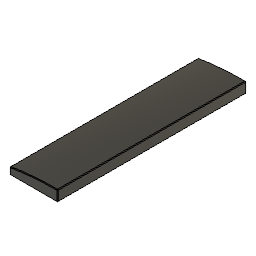
wrist_rest (Autodesk Fusion 360 design; units mm, degrees)
part number: 2026-06-30-23-31-08-090
Autodesk Fusion 360 part; units mm, degrees
sketch "Sketch1" plane through (0, 0, 0) normal (0, 0, 1) x (1, 0, 0)
  line L0 (0, 0) -> (78.5, 0)
  line L1 (0, 0) -> (0, 18)
  line L2 (78.5, 0) -> (78.5, 11.8)
  arc A0 (78.5, 11.8) -> (0, 18) centre (2.1231, -455.1742) ccw
  dimension "d3" = 78.5
  dimension "d4" = 18
  dimension "d5" = 11.8
  constraint coincident L0.start L1.start
  constraint horizontal L0
  constraint perpendicular L0 L1
  constraint perpendicular L0 L2
  measures "d3" distance of L0.start L0.end
  measures "d4" distance of L0.start L1.end
  measures "d5" distance of L0.end L2.end
extrude "Extrude1" add sketch "Sketch1" along normal blind 310
move_body "Move1" bodies 1 to x (1, 0, 0) y (0, 0, -1) z (0, 1, 0) at (0, 0, 0)
move_body "Move2" bodies 1 to x (-1, 0, 0) y (0, 1, 0) z (0, 0, -1) at (0, 0, 0)
sketch "Sketch3" plane through (0, 0, 0) normal (0, 0, -1) x (1, 0, 0)
  line L0 (0, 0) -> (-78.5, 0)
  line L1 (-78.5, 0) -> (-78.5, -310)
  line L2 (-78.5, -310) -> (0, -310)
  line L3 (0, -310) -> (0, 0)
  line L4 (-4, -306) -> (-4, -4)
  line L5 (-4, -4) -> (-74.5, -4)
  line L6 (-74.5, -4) -> (-74.5, -306)
  line L7 (-74.5, -306) -> (-4, -306)
  line L8 (-23.4372, -294.0415) -> (-16.4372, -298.0829)
  line L9 (-16.4372, -298.0829) -> (-9.4372, -294.0415)
  line L10 (-9.4372, -294.0415) -> (-9.4372, -285.9585)
  line L11 (-9.4372, -285.9585) -> (-16.4372, -281.9171)
  line L12 (-16.4372, -281.9171) -> (-23.4372, -285.9585)
  line L13 (-23.4372, -285.9585) -> (-23.4372, -294.0415)
  line L14 (-32.4372, -294.0415) -> (-32.4372, -285.9585)
  line L15 (-46.4372, -294.0415) -> (-39.4372, -298.0829)
  line L16 (-39.4372, -298.0829) -> (-32.4372, -294.0415)
  line L17 (-46.4372, -285.9585) -> (-46.4372, -294.0415)
  line L18 (-32.4372, -285.9585) -> (-39.4372, -281.9171)
  line L19 (-39.4372, -281.9171) -> (-46.4372, -285.9585)
  line L20 (-55.4372, -294.0415) -> (-55.4372, -285.9585)
  line L21 (-69.4372, -294.0415) -> (-62.4372, -298.0829)
  line L22 (-62.4372, -298.0829) -> (-55.4372, -294.0415)
  line L23 (-69.4372, -285.9585) -> (-69.4372, -294.0415)
  line L24 (-55.4372, -285.9585) -> (-62.4372, -281.9171)
  line L25 (-62.4372, -281.9171) -> (-69.4372, -285.9585)
  line L26 (-34.9913, -280.8853) -> (-27.9913, -284.9268)
  line L27 (-27.9913, -284.9268) -> (-20.9913, -280.8853)
  line L28 (-20.9913, -280.8853) -> (-20.9913, -272.8024)
  line L29 (-20.9913, -272.8024) -> (-27.9913, -268.761)
  line L30 (-27.9913, -268.761) -> (-34.9913, -272.8024)
  line L31 (-34.9913, -272.8024) -> (-34.9913, -280.8853)
  line L32 (-57.9913, -280.8853) -> (-50.9913, -284.9268)
  line L33 (-50.9913, -284.9268) -> (-43.9913, -280.8853)
  line L34 (-57.9913, -272.8024) -> (-57.9913, -280.8853)
  line L35 (-43.9913, -272.8024) -> (-50.9913, -268.761)
  line L36 (-43.9913, -280.8853) -> (-43.9913, -272.8024)
  line L37 (-50.9913, -268.761) -> (-57.9913, -272.8024)
  line L38 (-57.9913, -254.8853) -> (-50.9913, -258.9268)
  line L39 (-32.4372, -268.0415) -> (-32.4372, -259.9585)
  line L40 (-62.4372, -272.0829) -> (-55.4372, -268.0415)
  line L41 (-39.4372, -255.9171) -> (-46.4372, -259.9585)
  line L42 (-16.4372, -255.9171) -> (-23.4372, -259.9585)
  line L43 (-20.9913, -254.8853) -> (-20.9913, -246.8024)
  line L44 (-39.4372, -272.0829) -> (-32.4372, -268.0415)
  line L45 (-69.4372, -259.9585) -> (-69.4372, -268.0415)
  line L46 (-50.9913, -242.761) -> (-57.9913, -246.8024)
  line L47 (-23.4372, -268.0415) -> (-16.4372, -272.0829)
  line L48 (-46.4372, -259.9585) -> (-46.4372, -268.0415)
  line L49 (-16.4372, -272.0829) -> (-9.4372, -268.0415)
  line L50 (-57.9913, -246.8024) -> (-57.9913, -254.8853)
  line L51 (-55.4372, -268.0415) -> (-55.4372, -259.9585)
  line L52 (-62.4372, -255.9171) -> (-69.4372, -259.9585)
  line L53 (-9.4372, -259.9585) -> (-16.4372, -255.9171)
  line L54 (-55.4372, -259.9585) -> (-62.4372, -255.9171)
  line L55 (-50.9913, -258.9268) -> (-43.9913, -254.8853)
  line L56 (-34.9913, -246.8024) -> (-34.9913, -254.8853)
  line L57 (-43.9913, -254.8853) -> (-43.9913, -246.8024)
  line L58 (-23.4372, -259.9585) -> (-23.4372, -268.0415)
  line L59 (-46.4372, -268.0415) -> (-39.4372, -272.0829)
  line L60 (-34.9913, -254.8853) -> (-27.9913, -258.9268)
  line L61 (-43.9913, -246.8024) -> (-50.9913, -242.761)
  line L62 (-27.9913, -242.761) -> (-34.9913, -246.8024)
  line L63 (-27.9913, -258.9268) -> (-20.9913, -254.8853)
  line L64 (-20.9913, -246.8024) -> (-27.9913, -242.761)
  line L65 (-9.4372, -268.0415) -> (-9.4372, -259.9585)
  line L66 (-69.4372, -268.0415) -> (-62.4372, -272.0829)
  line L67 (-32.4372, -259.9585) -> (-39.4372, -255.9171)
  line L68 (-57.9913, -228.8853) -> (-50.9913, -232.9268)
  line L69 (-32.4372, -242.0415) -> (-32.4372, -233.9585)
  line L70 (-62.4372, -246.0829) -> (-55.4372, -242.0415)
  line L71 (-39.4372, -229.9171) -> (-46.4372, -233.9585)
  line L72 (-16.4372, -229.9171) -> (-23.4372, -233.9585)
  line L73 (-20.9913, -228.8853) -> (-20.9913, -220.8024)
  line L74 (-39.4372, -246.0829) -> (-32.4372, -242.0415)
  line L75 (-69.4372, -233.9585) -> (-69.4372, -242.0415)
  line L76 (-50.9913, -216.761) -> (-57.9913, -220.8024)
  line L77 (-23.4372, -242.0415) -> (-16.4372, -246.0829)
  line L78 (-46.4372, -233.9585) -> (-46.4372, -242.0415)
  line L79 (-16.4372, -246.0829) -> (-9.4372, -242.0415)
  line L80 (-57.9913, -220.8024) -> (-57.9913, -228.8853)
  line L81 (-55.4372, -242.0415) -> (-55.4372, -233.9585)
  line L82 (-62.4372, -229.9171) -> (-69.4372, -233.9585)
  line L83 (-9.4372, -233.9585) -> (-16.4372, -229.9171)
  line L84 (-55.4372, -233.9585) -> (-62.4372, -229.9171)
  line L85 (-50.9913, -232.9268) -> (-43.9913, -228.8853)
  line L86 (-34.9913, -220.8024) -> (-34.9913, -228.8853)
  line L87 (-43.9913, -228.8853) -> (-43.9913, -220.8024)
  line L88 (-23.4372, -233.9585) -> (-23.4372, -242.0415)
  line L89 (-46.4372, -242.0415) -> (-39.4372, -246.0829)
  line L90 (-34.9913, -228.8853) -> (-27.9913, -232.9268)
  line L91 (-43.9913, -220.8024) -> (-50.9913, -216.761)
  line L92 (-27.9913, -216.761) -> (-34.9913, -220.8024)
  line L93 (-27.9913, -232.9268) -> (-20.9913, -228.8853)
  line L94 (-20.9913, -220.8024) -> (-27.9913, -216.761)
  line L95 (-9.4372, -242.0415) -> (-9.4372, -233.9585)
  line L96 (-69.4372, -242.0415) -> (-62.4372, -246.0829)
  line L97 (-32.4372, -233.9585) -> (-39.4372, -229.9171)
  line L98 (-57.9913, -202.8853) -> (-50.9913, -206.9268)
  line L99 (-32.4372, -216.0415) -> (-32.4372, -207.9585)
  line L100 (-62.4372, -220.0829) -> (-55.4372, -216.0415)
  line L101 (-39.4372, -203.9171) -> (-46.4372, -207.9585)
  line L102 (-16.4372, -203.9171) -> (-23.4372, -207.9585)
  line L103 (-20.9913, -202.8853) -> (-20.9913, -194.8024)
  line L104 (-39.4372, -220.0829) -> (-32.4372, -216.0415)
  line L105 (-69.4372, -207.9585) -> (-69.4372, -216.0415)
  line L106 (-50.9913, -190.761) -> (-57.9913, -194.8024)
  line L107 (-23.4372, -216.0415) -> (-16.4372, -220.0829)
  line L108 (-46.4372, -207.9585) -> (-46.4372, -216.0415)
  line L109 (-16.4372, -220.0829) -> (-9.4372, -216.0415)
  line L110 (-57.9913, -194.8024) -> (-57.9913, -202.8853)
  line L111 (-55.4372, -216.0415) -> (-55.4372, -207.9585)
  line L112 (-62.4372, -203.9171) -> (-69.4372, -207.9585)
  line L113 (-9.4372, -207.9585) -> (-16.4372, -203.9171)
  line L114 (-55.4372, -207.9585) -> (-62.4372, -203.9171)
  line L115 (-50.9913, -206.9268) -> (-43.9913, -202.8853)
  line L116 (-34.9913, -194.8024) -> (-34.9913, -202.8853)
  line L117 (-43.9913, -202.8853) -> (-43.9913, -194.8024)
  line L118 (-23.4372, -207.9585) -> (-23.4372, -216.0415)
  line L119 (-46.4372, -216.0415) -> (-39.4372, -220.0829)
  line L120 (-34.9913, -202.8853) -> (-27.9913, -206.9268)
  line L121 (-43.9913, -194.8024) -> (-50.9913, -190.761)
  line L122 (-27.9913, -190.761) -> (-34.9913, -194.8024)
  line L123 (-27.9913, -206.9268) -> (-20.9913, -202.8853)
  line L124 (-20.9913, -194.8024) -> (-27.9913, -190.761)
  line L125 (-9.4372, -216.0415) -> (-9.4372, -207.9585)
  line L126 (-69.4372, -216.0415) -> (-62.4372, -220.0829)
  line L127 (-32.4372, -207.9585) -> (-39.4372, -203.9171)
  line L128 (-57.9913, -176.8853) -> (-50.9913, -180.9268)
  line L129 (-32.4372, -190.0415) -> (-32.4372, -181.9585)
  line L130 (-62.4372, -194.0829) -> (-55.4372, -190.0415)
  line L131 (-39.4372, -177.9171) -> (-46.4372, -181.9585)
  line L132 (-16.4372, -177.9171) -> (-23.4372, -181.9585)
  line L133 (-20.9913, -176.8853) -> (-20.9913, -168.8024)
  line L134 (-39.4372, -194.0829) -> (-32.4372, -190.0415)
  line L135 (-69.4372, -181.9585) -> (-69.4372, -190.0415)
  line L136 (-50.9913, -164.761) -> (-57.9913, -168.8024)
  line L137 (-23.4372, -190.0415) -> (-16.4372, -194.0829)
  line L138 (-46.4372, -181.9585) -> (-46.4372, -190.0415)
  line L139 (-16.4372, -194.0829) -> (-9.4372, -190.0415)
  line L140 (-57.9913, -168.8024) -> (-57.9913, -176.8853)
  line L141 (-55.4372, -190.0415) -> (-55.4372, -181.9585)
  line L142 (-62.4372, -177.9171) -> (-69.4372, -181.9585)
  line L143 (-9.4372, -181.9585) -> (-16.4372, -177.9171)
  line L144 (-55.4372, -181.9585) -> (-62.4372, -177.9171)
  line L145 (-50.9913, -180.9268) -> (-43.9913, -176.8853)
  line L146 (-34.9913, -168.8024) -> (-34.9913, -176.8853)
  line L147 (-43.9913, -176.8853) -> (-43.9913, -168.8024)
  line L148 (-23.4372, -181.9585) -> (-23.4372, -190.0415)
  line L149 (-46.4372, -190.0415) -> (-39.4372, -194.0829)
  line L150 (-34.9913, -176.8853) -> (-27.9913, -180.9268)
  line L151 (-43.9913, -168.8024) -> (-50.9913, -164.761)
  line L152 (-27.9913, -164.761) -> (-34.9913, -168.8024)
  line L153 (-27.9913, -180.9268) -> (-20.9913, -176.8853)
  line L154 (-20.9913, -168.8024) -> (-27.9913, -164.761)
  line L155 (-9.4372, -190.0415) -> (-9.4372, -181.9585)
  line L156 (-69.4372, -190.0415) -> (-62.4372, -194.0829)
  line L157 (-32.4372, -181.9585) -> (-39.4372, -177.9171)
  line L158 (-57.9913, -150.8853) -> (-50.9913, -154.9268)
  line L159 (-32.4372, -164.0415) -> (-32.4372, -155.9585)
  line L160 (-62.4372, -168.0829) -> (-55.4372, -164.0415)
  line L161 (-39.4372, -151.9171) -> (-46.4372, -155.9585)
  line L162 (-16.4372, -151.9171) -> (-23.4372, -155.9585)
  line L163 (-20.9913, -150.8853) -> (-20.9913, -142.8024)
  line L164 (-39.4372, -168.0829) -> (-32.4372, -164.0415)
  line L165 (-69.4372, -155.9585) -> (-69.4372, -164.0415)
  line L166 (-50.9913, -138.761) -> (-57.9913, -142.8024)
  line L167 (-23.4372, -164.0415) -> (-16.4372, -168.0829)
  line L168 (-46.4372, -155.9585) -> (-46.4372, -164.0415)
  line L169 (-16.4372, -168.0829) -> (-9.4372, -164.0415)
  line L170 (-57.9913, -142.8024) -> (-57.9913, -150.8853)
  line L171 (-55.4372, -164.0415) -> (-55.4372, -155.9585)
  line L172 (-62.4372, -151.9171) -> (-69.4372, -155.9585)
  line L173 (-9.4372, -155.9585) -> (-16.4372, -151.9171)
  line L174 (-55.4372, -155.9585) -> (-62.4372, -151.9171)
  line L175 (-50.9913, -154.9268) -> (-43.9913, -150.8853)
  line L176 (-34.9913, -142.8024) -> (-34.9913, -150.8853)
  line L177 (-43.9913, -150.8853) -> (-43.9913, -142.8024)
  line L178 (-23.4372, -155.9585) -> (-23.4372, -164.0415)
  line L179 (-46.4372, -164.0415) -> (-39.4372, -168.0829)
  line L180 (-34.9913, -150.8853) -> (-27.9913, -154.9268)
  line L181 (-43.9913, -142.8024) -> (-50.9913, -138.761)
  line L182 (-27.9913, -138.761) -> (-34.9913, -142.8024)
  line L183 (-27.9913, -154.9268) -> (-20.9913, -150.8853)
  line L184 (-20.9913, -142.8024) -> (-27.9913, -138.761)
  line L185 (-9.4372, -164.0415) -> (-9.4372, -155.9585)
  line L186 (-69.4372, -164.0415) -> (-62.4372, -168.0829)
  line L187 (-32.4372, -155.9585) -> (-39.4372, -151.9171)
  line L188 (-57.9913, -124.8853) -> (-50.9913, -128.9268)
  line L189 (-32.4372, -138.0415) -> (-32.4372, -129.9585)
  line L190 (-62.4372, -142.0829) -> (-55.4372, -138.0415)
  line L191 (-39.4372, -125.9171) -> (-46.4372, -129.9585)
  line L192 (-16.4372, -125.9171) -> (-23.4372, -129.9585)
  line L193 (-20.9913, -124.8853) -> (-20.9913, -116.8024)
  line L194 (-39.4372, -142.0829) -> (-32.4372, -138.0415)
  line L195 (-69.4372, -129.9585) -> (-69.4372, -138.0415)
  line L196 (-50.9913, -112.761) -> (-57.9913, -116.8024)
  line L197 (-23.4372, -138.0415) -> (-16.4372, -142.0829)
  line L198 (-46.4372, -129.9585) -> (-46.4372, -138.0415)
  line L199 (-16.4372, -142.0829) -> (-9.4372, -138.0415)
  line L200 (-57.9913, -116.8024) -> (-57.9913, -124.8853)
  line L201 (-55.4372, -138.0415) -> (-55.4372, -129.9585)
  line L202 (-62.4372, -125.9171) -> (-69.4372, -129.9585)
  line L203 (-9.4372, -129.9585) -> (-16.4372, -125.9171)
  line L204 (-55.4372, -129.9585) -> (-62.4372, -125.9171)
  line L205 (-50.9913, -128.9268) -> (-43.9913, -124.8853)
  line L206 (-34.9913, -116.8024) -> (-34.9913, -124.8853)
  line L207 (-43.9913, -124.8853) -> (-43.9913, -116.8024)
  line L208 (-23.4372, -129.9585) -> (-23.4372, -138.0415)
  line L209 (-46.4372, -138.0415) -> (-39.4372, -142.0829)
  line L210 (-34.9913, -124.8853) -> (-27.9913, -128.9268)
  line L211 (-43.9913, -116.8024) -> (-50.9913, -112.761)
  line L212 (-27.9913, -112.761) -> (-34.9913, -116.8024)
  line L213 (-27.9913, -128.9268) -> (-20.9913, -124.8853)
  line L214 (-20.9913, -116.8024) -> (-27.9913, -112.761)
  line L215 (-9.4372, -138.0415) -> (-9.4372, -129.9585)
  line L216 (-69.4372, -138.0415) -> (-62.4372, -142.0829)
  line L217 (-32.4372, -129.9585) -> (-39.4372, -125.9171)
  line L218 (-57.9913, -98.8853) -> (-50.9913, -102.9268)
  line L219 (-32.4372, -112.0415) -> (-32.4372, -103.9585)
  line L220 (-62.4372, -116.0829) -> (-55.4372, -112.0415)
  line L221 (-39.4372, -99.9171) -> (-46.4372, -103.9585)
  line L222 (-16.4372, -99.9171) -> (-23.4372, -103.9585)
  line L223 (-20.9913, -98.8853) -> (-20.9913, -90.8024)
  line L224 (-39.4372, -116.0829) -> (-32.4372, -112.0415)
  line L225 (-69.4372, -103.9585) -> (-69.4372, -112.0415)
  line L226 (-50.9913, -86.761) -> (-57.9913, -90.8024)
  line L227 (-23.4372, -112.0415) -> (-16.4372, -116.0829)
  line L228 (-46.4372, -103.9585) -> (-46.4372, -112.0415)
  line L229 (-16.4372, -116.0829) -> (-9.4372, -112.0415)
  line L230 (-57.9913, -90.8024) -> (-57.9913, -98.8853)
  line L231 (-55.4372, -112.0415) -> (-55.4372, -103.9585)
  line L232 (-62.4372, -99.9171) -> (-69.4372, -103.9585)
  line L233 (-9.4372, -103.9585) -> (-16.4372, -99.9171)
  line L234 (-55.4372, -103.9585) -> (-62.4372, -99.9171)
  line L235 (-50.9913, -102.9268) -> (-43.9913, -98.8853)
  line L236 (-34.9913, -90.8024) -> (-34.9913, -98.8853)
  line L237 (-43.9913, -98.8853) -> (-43.9913, -90.8024)
  line L238 (-23.4372, -103.9585) -> (-23.4372, -112.0415)
  line L239 (-46.4372, -112.0415) -> (-39.4372, -116.0829)
  line L240 (-34.9913, -98.8853) -> (-27.9913, -102.9268)
  line L241 (-43.9913, -90.8024) -> (-50.9913, -86.761)
  line L242 (-27.9913, -86.761) -> (-34.9913, -90.8024)
  line L243 (-27.9913, -102.9268) -> (-20.9913, -98.8853)
  line L244 (-20.9913, -90.8024) -> (-27.9913, -86.761)
  line L245 (-9.4372, -112.0415) -> (-9.4372, -103.9585)
  line L246 (-69.4372, -112.0415) -> (-62.4372, -116.0829)
  line L247 (-32.4372, -103.9585) -> (-39.4372, -99.9171)
  line L248 (-57.9913, -72.8853) -> (-50.9913, -76.9268)
  line L249 (-32.4372, -86.0415) -> (-32.4372, -77.9585)
  line L250 (-62.4372, -90.0829) -> (-55.4372, -86.0415)
  line L251 (-39.4372, -73.9171) -> (-46.4372, -77.9585)
  line L252 (-16.4372, -73.9171) -> (-23.4372, -77.9585)
  line L253 (-20.9913, -72.8853) -> (-20.9913, -64.8024)
  line L254 (-39.4372, -90.0829) -> (-32.4372, -86.0415)
  line L255 (-69.4372, -77.9585) -> (-69.4372, -86.0415)
  line L256 (-50.9913, -60.761) -> (-57.9913, -64.8024)
  line L257 (-23.4372, -86.0415) -> (-16.4372, -90.0829)
  line L258 (-46.4372, -77.9585) -> (-46.4372, -86.0415)
  line L259 (-16.4372, -90.0829) -> (-9.4372, -86.0415)
  line L260 (-57.9913, -64.8024) -> (-57.9913, -72.8853)
  line L261 (-55.4372, -86.0415) -> (-55.4372, -77.9585)
  line L262 (-62.4372, -73.9171) -> (-69.4372, -77.9585)
  line L263 (-9.4372, -77.9585) -> (-16.4372, -73.9171)
  line L264 (-55.4372, -77.9585) -> (-62.4372, -73.9171)
  line L265 (-50.9913, -76.9268) -> (-43.9913, -72.8853)
  line L266 (-34.9913, -64.8024) -> (-34.9913, -72.8853)
  line L267 (-43.9913, -72.8853) -> (-43.9913, -64.8024)
  line L268 (-23.4372, -77.9585) -> (-23.4372, -86.0415)
  line L269 (-46.4372, -86.0415) -> (-39.4372, -90.0829)
  line L270 (-34.9913, -72.8853) -> (-27.9913, -76.9268)
  line L271 (-43.9913, -64.8024) -> (-50.9913, -60.761)
  line L272 (-27.9913, -60.761) -> (-34.9913, -64.8024)
  line L273 (-27.9913, -76.9268) -> (-20.9913, -72.8853)
  line L274 (-20.9913, -64.8024) -> (-27.9913, -60.761)
  line L275 (-9.4372, -86.0415) -> (-9.4372, -77.9585)
  line L276 (-69.4372, -86.0415) -> (-62.4372, -90.0829)
  line L277 (-32.4372, -77.9585) -> (-39.4372, -73.9171)
  line L278 (-57.9913, -46.8853) -> (-50.9913, -50.9268)
  line L279 (-32.4372, -60.0415) -> (-32.4372, -51.9585)
  line L280 (-62.4372, -64.0829) -> (-55.4372, -60.0415)
  line L281 (-39.4372, -47.9171) -> (-46.4372, -51.9585)
  line L282 (-16.4372, -47.9171) -> (-23.4372, -51.9585)
  line L283 (-20.9913, -46.8853) -> (-20.9913, -38.8024)
  line L284 (-39.4372, -64.0829) -> (-32.4372, -60.0415)
  line L285 (-69.4372, -51.9585) -> (-69.4372, -60.0415)
  line L286 (-50.9913, -34.761) -> (-57.9913, -38.8024)
  line L287 (-23.4372, -60.0415) -> (-16.4372, -64.0829)
  line L288 (-46.4372, -51.9585) -> (-46.4372, -60.0415)
  line L289 (-16.4372, -64.0829) -> (-9.4372, -60.0415)
  line L290 (-57.9913, -38.8024) -> (-57.9913, -46.8853)
  line L291 (-55.4372, -60.0415) -> (-55.4372, -51.9585)
  line L292 (-62.4372, -47.9171) -> (-69.4372, -51.9585)
  line L293 (-9.4372, -51.9585) -> (-16.4372, -47.9171)
  line L294 (-55.4372, -51.9585) -> (-62.4372, -47.9171)
  line L295 (-50.9913, -50.9268) -> (-43.9913, -46.8853)
  line L296 (-34.9913, -38.8024) -> (-34.9913, -46.8853)
  line L297 (-43.9913, -46.8853) -> (-43.9913, -38.8024)
  line L298 (-23.4372, -51.9585) -> (-23.4372, -60.0415)
  line L299 (-46.4372, -60.0415) -> (-39.4372, -64.0829)
  line L300 (-34.9913, -46.8853) -> (-27.9913, -50.9268)
  line L301 (-43.9913, -38.8024) -> (-50.9913, -34.761)
  line L302 (-27.9913, -34.761) -> (-34.9913, -38.8024)
  line L303 (-27.9913, -50.9268) -> (-20.9913, -46.8853)
  line L304 (-20.9913, -38.8024) -> (-27.9913, -34.761)
  line L305 (-9.4372, -60.0415) -> (-9.4372, -51.9585)
  line L306 (-69.4372, -60.0415) -> (-62.4372, -64.0829)
  line L307 (-32.4372, -51.9585) -> (-39.4372, -47.9171)
  line L308 (-57.9913, -20.8853) -> (-50.9913, -24.9268)
  line L309 (-32.4372, -34.0415) -> (-32.4372, -25.9585)
  line L310 (-62.4372, -38.0829) -> (-55.4372, -34.0415)
  line L311 (-39.4372, -21.9171) -> (-46.4372, -25.9585)
  line L312 (-16.4372, -21.9171) -> (-23.4372, -25.9585)
  line L313 (-20.9913, -20.8853) -> (-20.9913, -12.8024)
  line L314 (-39.4372, -38.0829) -> (-32.4372, -34.0415)
  line L315 (-69.4372, -25.9585) -> (-69.4372, -34.0415)
  line L316 (-50.9913, -8.761) -> (-57.9913, -12.8024)
  line L317 (-23.4372, -34.0415) -> (-16.4372, -38.0829)
  line L318 (-46.4372, -25.9585) -> (-46.4372, -34.0415)
  line L319 (-16.4372, -38.0829) -> (-9.4372, -34.0415)
  line L320 (-57.9913, -12.8024) -> (-57.9913, -20.8853)
  line L321 (-55.4372, -34.0415) -> (-55.4372, -25.9585)
  line L322 (-62.4372, -21.9171) -> (-69.4372, -25.9585)
  line L323 (-9.4372, -25.9585) -> (-16.4372, -21.9171)
  line L324 (-55.4372, -25.9585) -> (-62.4372, -21.9171)
  line L325 (-50.9913, -24.9268) -> (-43.9913, -20.8853)
  line L326 (-34.9913, -12.8024) -> (-34.9913, -20.8853)
  line L327 (-43.9913, -20.8853) -> (-43.9913, -12.8024)
  line L328 (-23.4372, -25.9585) -> (-23.4372, -34.0415)
  line L329 (-46.4372, -34.0415) -> (-39.4372, -38.0829)
  line L330 (-34.9913, -20.8853) -> (-27.9913, -24.9268)
  line L331 (-43.9913, -12.8024) -> (-50.9913, -8.761)
  line L332 (-27.9913, -8.761) -> (-34.9913, -12.8024)
  line L333 (-27.9913, -24.9268) -> (-20.9913, -20.8853)
  line L334 (-20.9913, -12.8024) -> (-27.9913, -8.761)
  line L335 (-9.4372, -34.0415) -> (-9.4372, -25.9585)
  line L336 (-69.4372, -34.0415) -> (-62.4372, -38.0829)
  line L337 (-32.4372, -25.9585) -> (-39.4372, -21.9171)
  point P0 (-16.4372, -290)
  point P1 (-39.4372, -290)
  point P2 (-62.4372, -290)
  point P3 (-27.9913, -276.8439)
  point P4 (-50.9913, -276.8439)
  point P5 (-50.9913, -250.8439)
  point P6 (-62.4372, -264)
  point P7 (-39.4372, -264)
  point P8 (-27.9913, -250.8439)
  point P9 (-16.4372, -264)
  point P10 (-50.9913, -224.8439)
  point P11 (-62.4372, -238)
  point P12 (-39.4372, -238)
  point P13 (-27.9913, -224.8439)
  point P14 (-16.4372, -238)
  point P15 (-50.9913, -198.8439)
  point P16 (-62.4372, -212)
  point P17 (-39.4372, -212)
  point P18 (-27.9913, -198.8439)
  point P19 (-16.4372, -212)
  point P20 (-50.9913, -172.8439)
  point P21 (-62.4372, -186)
  point P22 (-39.4372, -186)
  point P23 (-27.9913, -172.8439)
  point P24 (-16.4372, -186)
  point P25 (-50.9913, -146.8439)
  point P26 (-62.4372, -160)
  point P27 (-39.4372, -160)
  point P28 (-27.9913, -146.8439)
  point P29 (-16.4372, -160)
  point P30 (-50.9913, -120.8439)
  point P31 (-62.4372, -134)
  point P32 (-39.4372, -134)
  point P33 (-27.9913, -120.8439)
  point P34 (-16.4372, -134)
  point P35 (-50.9913, -94.8439)
  point P36 (-62.4372, -108)
  point P37 (-39.4372, -108)
  point P38 (-27.9913, -94.8439)
  point P39 (-16.4372, -108)
  point P40 (-50.9913, -68.8439)
  point P41 (-62.4372, -82)
  point P42 (-39.4372, -82)
  point P43 (-27.9913, -68.8439)
  point P44 (-16.4372, -82)
  point P45 (-50.9913, -42.8439)
  point P46 (-62.4372, -56)
  point P47 (-39.4372, -56)
  point P48 (-27.9913, -42.8439)
  point P49 (-16.4372, -56)
  point P50 (-50.9913, -16.8439)
  point P51 (-62.4372, -30)
  point P52 (-39.4372, -30)
  point P53 (-27.9913, -16.8439)
  point P54 (-16.4372, -30)
  dimension "d59" = -4
  dimension "d60" = 7
  dimension "d63" = -23
  dimension "d64" = 0
  dimension "d65" = 7
  dimension "d66" = 7
  dimension "d69" = 0
  dimension "d70" = 260
  measures "d60" distance of P0 L13
  measures "d65" distance of P3 L31
  measures "d66" distance of P4 L34
extrude "Extrude2" cut sketch "Sketch3" against normal blind 8.8 contours L8 L9 L10 L11 L12 L13 | L14 L15 L16 L17 L18 L19 | L20 L21 L22 L23 L24 L25 | L26 L27 L28 L29 L30 L31 | L32 L33 L34 L35 L36 L37 | L38 L46 L50 L55 L57 L61 | L39 L41 L44 L48 L59 L67 | L40 L45 L51 L52 L54 L66 | L42 L47 L49 L53 L58 L65 | L43 L56 L60 L62 L63 L64 | L68 L76 L80 L85 L87 L91 | L69 L71 L74 L78 L89 L97 | L70 L75 L81 L82 L84 L96 | L72 L77 L79 L83 L88 L95 | L73 L86 L90 L92 L93 L94 | L98 L106 L110 L115 L117 L121 | L99 L101 L104 L108 L119 L127 | L100 L105 L111 L112 L114 L126 | L102 L107 L109 L113 L118 L125 | L103 L116 L120 L122 L123 L124 | L128 L136 L140 L145 L147 L151 | L129 L131 L134 L138 L149 L157 | L130 L135 L141 L142 L144 L156 | L132 L137 L139 L143 L148 L155 | L133 L146 L150 L152 L153 L154 | L158 L166 L170 L175 L177 L181 | L159 L161 L164 L168 L179 L187 | L160 L165 L171 L172 L174 L186 | L162 L167 L169 L173 L178 L185 | L163 L176 L180 L182 L183 L184 | L188 L196 L200 L205 L207 L211 | L189 L191 L194 L198 L209 L217 | L190 L195 L201 L202 L204 L216 | L192 L197 L199 L203 L208 L215 | L193 L206 L210 L212 L213 L214 | L218 L226 L230 L235 L237 L241 | L219 L221 L224 L228 L239 L247 | L220 L225 L231 L232 L234 L246 | L222 L227 L229 L233 L238 L245 | L223 L236 L240 L242 L243 L244 | L248 L256 L260 L265 L267 L271 | L249 L251 L254 L258 L269 L277 | L250 L255 L261 L262 L264 L276 | L252 L257 L259 L263 L268 L275 | L253 L266 L270 L272 L273 L274 | L278 L286 L290 L295 L297 L301 | L279 L281 L284 L288 L299 L307 | L280 L285 L291 L292 L294 L306 | L282 L287 L289 L293 L298 L305 | L283 L296 L300 L302 L303 L304 | L308 L316 L320 L325 L327 L331 | L309 L311 L314 L318 L329 L337 | L310 L315 L321 L322 L324 L336 | L312 L317 L319 L323 L328 L335 | L313 L326 L330 L332 L333 L334
fillet "Fillet1" radius 1 1 edges at (-78.5, 155, 11.8)
fillet "Fillet2" radius 1 1 edges at (-78.5, 155, 0)
fillet "Fillet3" radius 1 5 edges at (-38.75, 0, 0) (-78.2071, 0, 0.2929) (-78.5, 0, 5.9747) (-78.2615, 0, 11.5977) (-38.9548, 0, 16.5691)
fillet "Fillet4" radius 1 5 edges at (0, 155.5, 0) (0, 0.2929, 0.2929) (0, 0, 9) (0, 0.2929, 17.7071) (0, 155.5, 18)
fillet "Fillet5" radius 1 8 edges at (-0.2921, 310, 17.7097) (0, 310, 9.0017) (-0.2929, 310, 0.2929) (-39.25, 310, 0) (-78.2071, 310, 0.2929) (-78.5, 310, 5.9747) (-78.2615, 310, 11.5977) (-39.4521, 310, 16.53)
